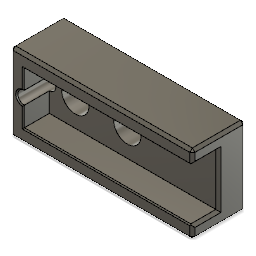
_beam drill guide.ea70630a-8385-41b1-85d9-3c377456444a (Autodesk Fusion 360 design; units mm, degrees)
Autodesk Fusion 360 part; units mm, degrees
sketch "Sketch1" plane through (0, 0, 0) normal (0, 0, 1) x (1, 0, 0)
  circle A0 centre (0, 0) radius 5.25
  line L0 (0, 0) -> (20, 0)
  circle A1 centre (20, 0) radius 5.25
  line L1 (0, 0) -> (-15, 0)
  line L2 (-15, 0) -> (-15, 15)
  line L3 (-15, 0) -> (-15, -15)
  line L4 (-15, -15) -> (55, -15)
  line L5 (-15, 15) -> (55, 15)
  line L6 (55, 15) -> (55, -15)
  circle A2 centre (-10, 0) radius 2.5
  dimension "d1" = 10.5
  dimension "d2" = 20
  dimension "d3" = 10.5
  dimension "d4" = 15
  dimension "d5" = 15
  dimension "d6" = 15
  dimension "d7" = 70
  dimension "d8" = 5
  constraint coincident A0.centre L0.start
  constraint horizontal L0
  constraint coincident L0.end A1.centre
  constraint parallel L0 L1
  constraint perpendicular L1 L2
  constraint perpendicular L1 L3
  constraint perpendicular L3 L4
  constraint perpendicular L2 L5
  constraint perpendicular L5 L6
  constraint coincident L1 A2.centre
  measures "d1" diameter of A0
  measures "d2" distance of A0.centre L0.end
  measures "d3" diameter of A1
  measures "d4" distance of A0.centre L1.end
  measures "d5" distance of L1.end L2.end
  measures "d6" distance of L1.end L3.end
  measures "d7" distance of L3.end L4.end
  measures "d8" diameter of A2
extrude "Extrude1" add sketch "Sketch1" along normal blind 8.5
sketch "Sketch2" plane through (0, 0, 8.5) normal (0, 0, 1) x (1, 0, 0)
  circle A0 centre (0, 0) radius 5.25
  circle A1 centre (-10, 0) radius 2.5
  circle A2 centre (20, 0) radius 5.25
  line L0 (-15, 15) -> (-15, -15)
  line L1 (-15, -15) -> (55, -15)
  line L2 (55, -15) -> (55, 15)
  line L3 (55, 15) -> (-15, 15)
  line L4 (-10, 10) -> (55, 10)
  line L5 (55, 10) -> (55, -10)
  line L6 (55, -10) -> (-10, -10)
  line L7 (-10, -10) -> (-10, 10)
  dimension "d11" = 20
  dimension "d12" = 65
  constraint horizontal L4
  constraint vertical L5
  constraint horizontal L6
  constraint vertical L7
  measures "d11" distance of L4.start L6.end
  measures "d12" distance of L4.start L4.end
extrude "Extrude2" add sketch "Sketch2" along normal blind 10 contours A1 L0 L1 L2 L3 L4 L6 L7
sketch "Sketch3" plane through (0, 0, 0) normal (0, 0, -1) x (-1, 0, 0)
  circle A0 centre (0, 0) radius 5.25
  circle A1 centre (10, 0) radius 2.5
  circle A2 centre (-20, 0) radius 5.25
  line L0 (15, -15) -> (15, 15)
  line L1 (15, 15) -> (-55, 15)
  line L2 (-55, 15) -> (-55, -15)
  line L3 (-55, -15) -> (15, -15)
  circle A3 centre (-20, 0) radius 7.25
  circle A4 centre (0, 0) radius 7.25
  dimension "d15" = 14.5
  dimension "d16" = 14.5
  constraint concentric A2 A3
  constraint concentric A0 A4
  measures "d15" diameter of A3
  measures "d16" diameter of A4
extrude "Extrude3" add sketch "Sketch3" along normal blind 2 contours L0 L1 L2 L3
chamfer "Chamfer1" distance 1 angle 45 16 edges at (20, 15, -2) (-15, 15, 8.25) (-15, 0, -2) (-15, -15, 8.25) (20, -15, -2) (55, 0, -2) (20, -15, 18.5) (-15, 0, 18.5) (20, 15, 18.5) (55, 15, 8.25) (55, -15, 8.25) (55, -12.5, 18.5) (55, 12.5, 18.5) (55, -10, 13.5) (55, 0, 8.5) (55, 10, 13.5)
chamfer "Chamfer2" distance 0.4 angle 45 5 edges at (22, -10, 18.5) (-10, -6.25, 18.5) (-12.5, 0, 18.5) (-10, 6.25, 18.5) (22, 10, 18.5)
